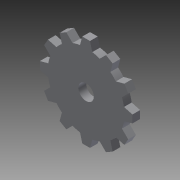
# Autodesk Inventor part: Sun
Saved by Autodesk Inventor 2013 (Build 170138000, 138)
## iProperties
Created: 2014-02-12
Part Number: Sun
Material: Generic
Document SubType Name: Modeling
Designer: robotics
Density: 1 g/cm^3
Author: robotics
Autodesk Inventor part; units mm, degrees
ref_plane "YZ Plane" through (0, 0, 0) normal (1, 0, 0) x (0, 1, 0)
ref_plane "XZ Plane" through (0, 0, 0) normal (0, 1, 0) x (-1, 0, 0)
ref_plane "XY Plane" through (0, 0, 0) normal (0, 0, 1) x (1, 0, 0)
sketch "Sketch2" plane through (0, 0, 0) normal (0, 0, 1) x (1, 0, 0)
  line L0 (0, 15.4964) -> (0, 0) construction
  line L1 (1.2621, 7.7771) -> (0.7937, 9.525)
  line L2 (0.7937, 9.525) -> (0, 9.525)
  line L3 (-1.2621, 7.7771) -> (-0.7937, 9.525)
  line L4 (-0.7937, 9.525) -> (0, 9.525)
  line L5 (-2.7955, 7.3662) -> (-4.0751, 8.6458)
  line L6 (-4.0751, 8.6458) -> (-4.7625, 8.2489)
  line L7 (-4.9815, 6.1041) -> (-5.4499, 7.852)
  line L8 (-5.4499, 7.852) -> (-4.7625, 8.2489)
  line L9 (-6.1041, 4.9815) -> (-7.852, 5.4499)
  line L10 (-7.852, 5.4499) -> (-8.2489, 4.7625)
  line L11 (-7.3662, 2.7955) -> (-8.6458, 4.0751)
  line L12 (-8.6458, 4.0751) -> (-8.2489, 4.7625)
  line L13 (-7.7771, 1.2621) -> (-9.525, 0.7938)
  line L14 (-9.525, 0.7938) -> (-9.525, 0)
  line L15 (-7.7771, -1.2621) -> (-9.525, -0.7937)
  line L16 (-9.525, -0.7937) -> (-9.525, 0)
  line L17 (-7.3662, -2.7955) -> (-8.6458, -4.0751)
  line L18 (-8.6458, -4.0751) -> (-8.2489, -4.7625)
  line L19 (-6.1041, -4.9815) -> (-7.852, -5.4499)
  line L20 (-7.852, -5.4499) -> (-8.2489, -4.7625)
  line L21 (-4.9815, -6.1041) -> (-5.4499, -7.852)
  line L22 (-5.4499, -7.852) -> (-4.7625, -8.2489)
  line L23 (-2.7955, -7.3662) -> (-4.0751, -8.6458)
  line L24 (-4.0751, -8.6458) -> (-4.7625, -8.2489)
  line L25 (-1.2621, -7.7771) -> (-0.7938, -9.525)
  line L26 (-0.7938, -9.525) -> (0, -9.525)
  line L27 (1.2621, -7.7771) -> (0.7937, -9.525)
  line L28 (0.7937, -9.525) -> (0, -9.525)
  line L29 (2.7955, -7.3662) -> (4.0751, -8.6458)
  line L30 (4.0751, -8.6458) -> (4.7625, -8.2489)
  line L31 (4.9815, -6.1041) -> (5.4499, -7.852)
  line L32 (5.4499, -7.852) -> (4.7625, -8.2489)
  line L33 (6.1041, -4.9815) -> (7.852, -5.4499)
  line L34 (7.852, -5.4499) -> (8.2489, -4.7625)
  line L35 (7.3662, -2.7955) -> (8.6458, -4.0751)
  line L36 (8.6458, -4.0751) -> (8.2489, -4.7625)
  line L37 (7.7771, -1.2621) -> (9.525, -0.7938)
  line L38 (9.525, -0.7938) -> (9.525, 0)
  line L39 (7.7771, 1.2621) -> (9.525, 0.7937)
  line L40 (9.525, 0.7937) -> (9.525, 0)
  line L41 (7.3662, 2.7955) -> (8.6458, 4.0751)
  line L42 (8.6458, 4.0751) -> (8.2489, 4.7625)
  line L43 (6.1041, 4.9815) -> (7.852, 5.4499)
  line L44 (7.852, 5.4499) -> (8.2489, 4.7625)
  line L45 (4.9815, 6.1041) -> (5.4499, 7.852)
  line L46 (5.4499, 7.852) -> (4.7625, 8.2489)
  line L47 (2.7955, 7.3662) -> (4.0751, 8.6458)
  line L48 (4.0751, 8.6458) -> (4.7625, 8.2489)
  line L49 (-2.7955, 7.3662) -> (-1.2621, 7.7771) construction
  line L50 (-0.7937, 9.525) -> (0.7937, 9.525) construction
  arc A0 (-1.2621, 7.7771) -> (-2.7955, 7.3662) centre (0, 0) ccw
  arc A1 (-4.9815, 6.1041) -> (-6.1041, 4.9815) centre (0, 0) ccw
  arc A2 (-7.3662, 2.7955) -> (-7.7771, 1.2621) centre (0, 0) ccw
  arc A3 (-7.7771, -1.2621) -> (-7.3662, -2.7955) centre (0, 0) ccw
  arc A4 (-6.1041, -4.9815) -> (-4.9815, -6.1041) centre (0, 0) ccw
  arc A5 (-2.7955, -7.3662) -> (-1.2621, -7.7771) centre (0, 0) ccw
  arc A6 (1.2621, -7.7771) -> (2.7955, -7.3662) centre (0, 0) ccw
  arc A7 (4.9815, -6.1041) -> (6.1041, -4.9815) centre (0, 0) ccw
  arc A8 (7.3662, -2.7955) -> (7.7771, -1.2621) centre (0, 0) ccw
  arc A9 (7.7771, 1.2621) -> (7.3662, 2.7955) centre (0, 0) ccw
  arc A10 (6.1041, 4.9815) -> (4.9815, 6.1041) centre (0, 0) ccw
  arc A11 (2.7955, 7.3662) -> (1.2621, 7.7771) centre (0, 0) ccw
  dimension "d5" = 1.5875
  dimension "d6" = 9.525
  dimension "d7" = 120
  constraints: 102 end point, 24 point on circle, 12 centre point, 2 symmetric about line, 1 coincident, 1 collinear, 1 equal length, 1 perpendicular, 1 point on line, 1 vertical, 109 other
  measures "d5" distance of L3.end L1.end
  measures "d6" distance of L0.end L2.end
  measures "d7" angle of L3 L49
extrude "Extrusion1" add sketch "Sketch2" along normal blind 1.5875
sketch "Sketch3" plane through (0, 0, 1.5875) normal (0, 0, 1) x (1, 0, 0)
  arc A0 (2.7955, 7.3662) -> (1.2621, 7.7771) centre (0, 0) ccw projected
  circle A1 centre (0, 0) radius 1.5875
  dimension "d10" = 3.175
  constraints: 1 centre point, 1 coincident
  measures "d10" diameter of A1
extrude "Extrusion2" cut sketch "Sketch3" against normal up to next
body "Solid1"
